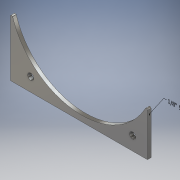
# Autodesk Inventor part: 1-8inch_Sieve_Piece1
Saved by Autodesk Inventor 2018 (Build 220112000, 112)
## iProperties
Created: 2018-01-22
Part Number: 1-8inch_Sieve_Piece1
Material: Generic
Document SubType Name: Modeling
Designer: Olivier
Density: 1 g/cm^3
Appearance: Default
Author: Olivier
Autodesk Inventor part; units mm, degrees
ref_plane "YZ Plane" through (0, 0, 0) normal (1, 0, 0) x (0, 1, 0)
ref_plane "XZ Plane" through (0, 0, 0) normal (0, 1, 0) x (-1, 0, 0)
ref_plane "XY Plane" through (0, 0, 0) normal (0, 0, 1) x (1, 0, 0)
sketch "Sketch1" plane through (0, 0, 0) normal (0, 0, 1) x (1, 0, 0)
  arc A0 (-17, -31.2731) -> (-18.866, -30.7731) centre (-18, -31.2731) ccw
  line L0 (-17, -31.2731) -> (-17, -69)
  line L1 (-17, -69) -> (-138, -69)
  line L2 (-138, -69) -> (-138, -19.5192)
  arc A1 (-136.0462, -19.2189) -> (-138, -19.5192) centre (-137, -19.5192) ccw
  arc A2 (-136.0462, -19.2189) -> (-19.5744, -32) centre (-75, 0) ccw
  line L3 (-19.5744, -32) -> (-18.866, -30.7731)
  circle A3 centre (-30, -57) radius 2.75
  circle A4 centre (-120, -57) radius 2.75
  line L4 (-138, -69) -> (-17, -69)
  arc A5 (-17, -31.2731) -> (-18.866, -30.7731) centre (-18, -31.2731) ccw
  line L5 (-17, -31.2731) -> (-17, -69)
  line L6 (-17, -69) -> (-138, -69)
  line L7 (-138, -69) -> (-138, -19.5192)
  arc A6 (-136.0462, -19.2189) -> (-138, -19.5192) centre (-137, -19.5192) ccw
  arc A7 (-136.0462, -19.2189) -> (-19.5744, -32) centre (-75, 0) ccw
  line L8 (-19.5744, -32) -> (-18.866, -30.7731)
  circle A8 centre (-30, -57) radius 2.75
  circle A9 centre (-120, -57) radius 2.75
  point P0 (0, 0)
  constraints: 18 end point, 12 point on circle, 10 centre point
extrude "Extrusion1" add sketch "Sketch1" along normal blind 3.175
body "Solid1"
